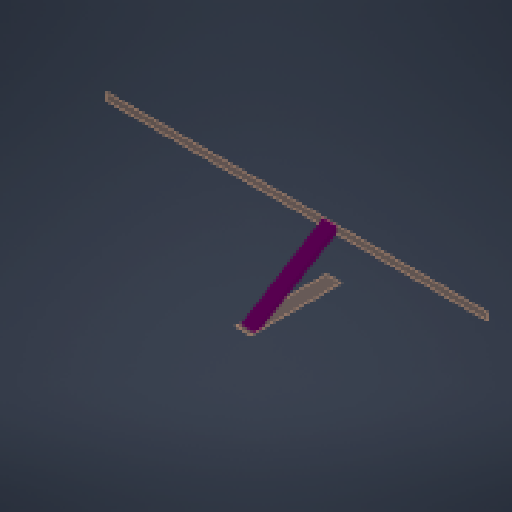
# Autodesk Inventor part: SideConnectors
Saved by Autodesk Inventor 2027 (Build 310192000, 192)
## iProperties
Created: 2026-08-07
Part Number: SideConnectors
Material: Generic
Document SubType Name: Modeling
Designer: lucas
Density: 1 g/cm^3
Appearance: Default
Author: lucas
Autodesk Inventor part; units mm, degrees
ref_plane "YZ Plane" through (0, 0, 0) normal (1, 0, 0) x (0, 1, 0)
ref_plane "XZ Plane" through (0, 0, 0) normal (0, 1, 0) x (-1, 0, 0)
ref_plane "XY Plane" through (0, 0, 0) normal (0, 0, 1) x (1, 0, 0)
ref_plane "Work Plane1" through (0, 0, 0) normal (0, 0, 1) x (1, 0, 0)
sketch "Sketch1" plane through (0, 0, 0) normal (0, 0, 1) x (1, 0, 0)
  line L0 (1473.2, 0) -> (1473.2, 50.8) projected
  line L1 (0, 50.8) -> (2565.4, 50.8) projected
  line L2 (1574.8, 0) -> (1574.8, 50.8) projected
  line L3 (1574.5938, 0) -> (1473.2, 0) projected
  line L4 (1473.2, 0) -> (1574.8, 0)
  line L5 (1574.8, 0) -> (1574.8, 50.8)
  line L6 (1574.8, 50.8) -> (1473.2, 50.8)
  line L7 (1473.2, 50.8) -> (1473.2, 0)
  point P0 (0, 0)
  constraints: 8 end point, 2 parallel, 1 horizontal, 1 perpendicular
ref_plane "Work Plane2" through (1524, -330.2, 304.8) normal (0, 1, 0) x (-1, 0, 0)
sketch "Sketch2" plane through (1524, -330.2, 304.8) normal (0, 1, 0) x (-1, 0, 0)
  line L0 (-50.5938, 254) -> (50.8, 254) projected
  line L1 (50.8, 203.2) -> (50.8, 304.8) projected
  line L2 (71.0788, 304.8) -> (-70.8726, 304.8)
  line L3 (-50.5938, 304.8) -> (-50.5938, 254) projected
  line L4 (50.8, 304.8) -> (-50.5938, 304.8)
  line L5 (-50.5938, 304.8) -> (-50.5938, 254)
  line L6 (-50.5938, 254) -> (50.8, 254)
  line L7 (50.8, 254) -> (50.8, 304.8)
  point P0 (1524, -304.8)
  constraints: 10 end point, 2 horizontal, 2 parallel, 1 perpendicular, 2 other
loft "Loft1" add profiles "Sketch2", "Sketch1"
body "Solid1"
